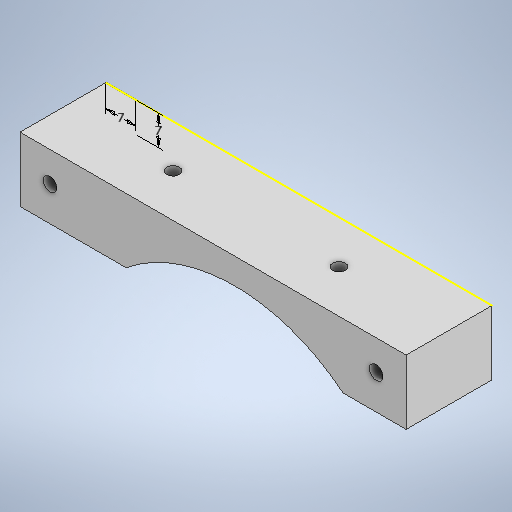
# Autodesk Inventor part: Base Ventilador
Saved by Autodesk Inventor 2025.2 (Build 292293000, 293)
## iProperties
Created: 2025-01-28
Part Number: Base Ventilador
Material: Genérico
Document SubType Name: Modeling
Designer: TUF GAMING F15
Density: 1 g/cm^3
Appearance: Valor por defecto
Author: TUF GAMING F15
Autodesk Inventor part; units mm, degrees
ref_plane "YZ Plane" through (0, 0, 0) normal (1, 0, 0) x (0, 1, 0)
ref_plane "XZ Plane" through (0, 0, 0) normal (0, 1, 0) x (-1, 0, 0)
ref_plane "XY Plane" through (0, 0, 0) normal (0, 0, 1) x (1, 0, 0)
sketch "Boceto1" plane through (0, 0, 0) normal (0, 1, 0) x (-1, 0, 0)
  line L0 (0, 0) -> (-80, 0)
  line L1 (-80, 0) -> (-80, -10)
  line L2 (-80, -10) -> (0, -10)
  line L3 (0, -10) -> (0, 0)
  line L4 (5, 0) -> (5, 5)
  line L5 (-80, -10) -> (-80, -15)
  line L6 (-80, -15) -> (-85, -15)
  line L7 (5, 5) -> (-85, 5)
  line L8 (-85, 5) -> (-85, -15)
  line L9 (-85, -15) -> (5, -15)
  line L10 (5, -15) -> (5, 5)
  dimension "d1" = 10
  dimension "d2" = 5
  dimension "d3" = 5
  dimension "d5" = 5
  constraints: 22 end point, 4 parallel, 3 perpendicular, 2 horizontal, 1 vertical
  measures "d1" distance of L1.end L0.end
  measures "d2" distance of L0.start L4.start
  measures "d3" distance of L4.start L4.end
  measures "d5" distance of L5.end L6.end
extrude "Extrusión1" add sketch "Boceto1" along normal blind 15
sketch "Boceto2" plane through (0, 15, 0) normal (0, 1, 0) x (1, 0, 0)
  line L0 (80, 10) -> (80, 0) projected
  line L1 (80, 0) -> (0, 0)
  line L2 (0, 0) -> (0, 10)
  line L3 (0, 10) -> (80, 10)
  line L4 (80, 10) -> (80, 0)
  constraints: 8 end point, 2 parallel, 1 horizontal, 1 perpendicular
extrude "Extrusión2" add sketch "Boceto2" against normal blind 5
sketch "Boceto3" plane through (-5, 0, 5) normal (0, 0, 1) x (1, 0, 0)
  line L0 (90, 15) -> (90, 9)
  line L1 (90, 0) -> (90, 15) projected
  line L2 (90, 9) -> (50, 9)
  line L3 (50, 9) -> (50, -31)
  circle A0 centre (50, -31) radius 40
  point P0 (5, 0)
  dimension "d10" = 6
  dimension "d11" = 40
  dimension "d12" = 40
  constraints: 6 end point, 1 coincident, 1 perpendicular, 1 point on line, 1 vertical, 1 vertical alignment, 2 other
  measures "d10" distance of L0.start L0.end
  measures "d11" distance of L0.end L2.end
  measures "d12" distance of L2.end L3.end
extrude "Extrusión3" cut sketch "Boceto3" against normal blind 21
sketch "Boceto4" plane through (0, 10, 0) normal (0, -1, 0) x (1, 0, 0)
  line L0 (0, 0) -> (0, -5)
  line L1 (0, 0) -> (0, -10) projected
  line L2 (0, -5) -> (80, -5)
  line L3 (80, -10) -> (80, 0) projected
  line L4 (80, -5) -> (59.34, -5)
  line L5 (0, -5) -> (20.66, -5)
  dimension "d15" = 5
  dimension "d16" = 20.66
  dimension "d17" = 20.66
  constraints: 8 end point, 2 midpoint, 2 point on line
  measures "d15" distance of L0.start L0.end
  measures "d16" distance of L2.end L4.end
  measures "d17" distance of L0.end L5.end
hole "Agujero1" at (20.66, 10, -5) at (59.34, 10, -5) direction (0, 1, 0) diameter 3 end through all countersink diameter 5 countersink angle 90
sketch "Boceto5" plane through (85, 15, -15) normal (0, 0, -1) x (-1, 0, 0)
  line L0 (90, -15) -> (90, 0) projected
  line L1 (90, 0) -> (83, 0)
  line L2 (0, 0) -> (90, 0) projected
  line L3 (83, 0) -> (83, -7)
  point P0 (85, -15)
  dimension "d25" = 7
  dimension "d26" = 7
  constraints: 4 end point, 1 perpendicular, 1 point on line
  measures "d25" distance of L0.end L1.end
  measures "d26" distance of L1.end L3.end
sketch "Boceto6" plane through (85, 15, -15) normal (0, 0, -1) x (-1, 0, 0)
  line L0 (0, 0) -> (90, 0) projected
  line L1 (0, 0) -> (0, -7)
  line L2 (0, -15) -> (0, 0) projected
  line L3 (0, -7) -> (7, -7)
  circle A0 centre (7, -7) radius 1.6
  line L4 (90, 0) -> (83, 0)
  line L5 (83, 0) -> (83, -7)
  circle A1 centre (83, -7) radius 1.6
  point P0 (85, -15)
  dimension "d27" = 7
  dimension "d28" = 7
  dimension "d29" = 3.2
  dimension "d30" = 7
  dimension "d31" = 7
  dimension "d32" = 3.2
  constraints: 8 end point, 2 centre point, 2 coincident, 2 perpendicular, 2 point on line
  measures "d27" distance of L0.start L1.end
  measures "d28" distance of L1.end L3.end
  measures "d29" diameter of A0
  measures "d30" distance of L0.end L4.end
  measures "d31" distance of L4.end L5.end
  measures "d32" diameter of A1
extrude "Extrusión4" cut sketch "Boceto6" against normal blind 28.75
